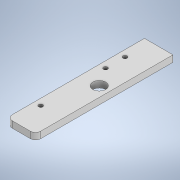
# Autodesk Inventor part: upper plate slide
Saved by Autodesk Inventor 2021 (Build 250183000, 183)
## iProperties
Created: 2020-09-03
Part Number: upper plate slide
Material: Generic
Document SubType Name: Modeling
Designer: jgray
Density: 1 g/cm^3
Appearance: Default
Author: jgray
Autodesk Inventor part; units mm, degrees
ref_plane "YZ Plane" through (0, 0, 0) normal (1, 0, 0) x (0, 1, 0)
ref_plane "XZ Plane" through (0, 0, 0) normal (0, 1, 0) x (-1, 0, 0)
ref_plane "XY Plane" through (0, 0, 0) normal (0, 0, 1) x (1, 0, 0)
sketch "Sketch1" plane through (0, 0, 0) normal (0, 1, 0) x (-1, 0, 0)
  line L0 (4, 0) -> (18, 0)
  line L1 (22, -4) -> (22, -106)
  line L2 (22, -106) -> (0, -106)
  line L3 (0, -106) -> (0, -4)
  arc A0 (22, -4) -> (18, 0) centre (18, -4) ccw
  arc A1 (4, 0) -> (0, -4) centre (4, -4) ccw
  point P0 (0, 0)
  point P1 (22, 0)
  dimension "d0" = 22
  dimension "d1" = 106
  dimension "d2" = 4
  constraints: 8 end point, 4 point on circle, 4 point on line, 4 tangent, 2 centre point, 2 parallel, 1 equal radius, 1 horizontal, 1 perpendicular
  measures "d0" distance of L1.end L2.end
  measures "d1" distance of point (22, 0) L1.end
  measures "d2" radius of A0
extrude "Extrusion1" add sketch "Sketch1" along normal blind 5
sketch "Sketch2" plane through (0, 5, 0) normal (0, 1, 0) x (1, 0, 0)
  line L0 (-7.75, -15.5804) -> (-7.75, 135.2593) construction
  line L1 (0, 4) -> (0, 106) construction
  line L2 (0, 106) -> (-22, 106) projected
  point P0 (0, 0)
  point P1 (-7.75, 56.9)
  dimension "d5" = 7.75
  dimension "d6" = 49.1
  constraints: 2 end point, 1 point on line, 1 vertical
  measures "d5" distance between parallel lines of L1 L0
  measures "d6" distance from line of L2 point (-7.75, 56.9)
hole "Hole1" at (-7.75, 5, -56.9) direction (0, -1, 0) diameter 10 end through all
sketch "Sketch3" plane through (0, 5, 0) normal (0, 1, 0) x (1, 0, 0)
  line L0 (-17, -17.788) -> (-17, 124.5417) construction
  line L1 (0, 4) -> (0, 106) construction
  line L2 (0, 106) -> (-22, 106) construction
  line L3 (0, 106) -> (-22, 106) construction
  point P0 (0, 0)
  point P1 (-17, 86)
  point P2 (-17, 21)
  point P3 (-17, 71)
  dimension "d14" = 17
  dimension "d15" = 20
  dimension "d16" = 35
  dimension "d17" = 85
  constraints: 3 point on line, 2 end point, 1 vertical
  measures "d14" distance between parallel lines of L1 L0
  measures "d15" distance from line of L2 point (-17, 86)
  measures "d16" distance from line of point (-17, 71) L2
  measures "d17" distance from line of point (-17, 21) L2
hole "Hole2" at (-17, 5, -86) at (-17, 5, -21) at (-17, 5, -71) direction (0, -1, 0) diameter 3.2 end through all
body "Solid1"
